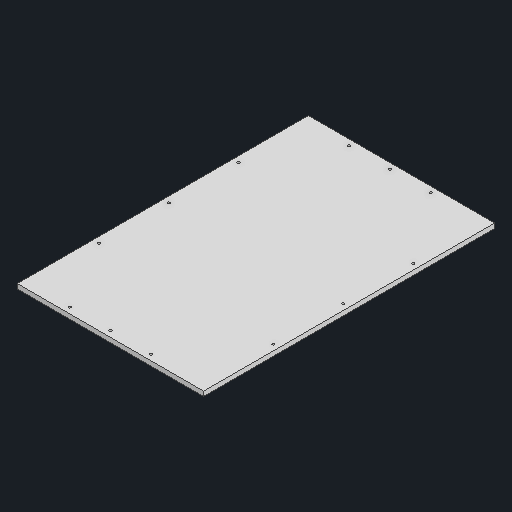
# Autodesk Inventor part: TeflonPlate
Saved by Autodesk Inventor 2027 (Build 310192060, 192F)
## iProperties
Created: 2026-06-12
Part Number: TeflonPlate
Material: Generic
Document SubType Name: Modeling
Designer: kw
Density: 1 g/cm^3
Appearance: Default
Author: kw
Autodesk Inventor part; units mm, degrees
ref_plane "YZ Plane" through (0, 0, 0) normal (1, 0, 0) x (0, 1, 0)
ref_plane "XZ Plane" through (0, 0, 0) normal (0, 1, 0) x (-1, 0, 0)
ref_plane "XY Plane" through (0, 0, 0) normal (0, 0, 1) x (1, 0, 0)
sketch "Sketch1" plane through (0, 0, 0) normal (0, 1, 0) x (-1, 0, 0)
  line L0 (0, 0) -> (-300, 0)
  line L1 (-300, 0) -> (-300, -500)
  line L2 (-300, -500) -> (0, -500)
  line L3 (0, -500) -> (0, 0)
  line L4 (-300, -500) -> (-320, -500)
  line L5 (-320, -500) -> (-320, 0)
  line L6 (-320, 0) -> (-300, 0)
  line L7 (-300, 0) -> (-300, -500)
  dimension "d101" = 300
  dimension "d102" = 500
  dimension "d110" = 20
  constraints: 16 end point, 4 parallel, 2 horizontal, 2 perpendicular
  measures "d101" distance of L2.end L1.end
  measures "d102" distance of L1.end L0.end
  measures "d110" distance of L5.end L6.end
extrude "Extrusion1" add sketch "Sketch1" along normal blind 8
sketch "Sketch4" plane through (0, 8, 0) normal (0, 1, 0) x (1, 0, 0)
  circle A0 centre (80, 490) radius 2.15 projected
  circle A1 centre (150, 490) radius 2.15 projected
  circle A2 centre (220, 490) radius 2.15 projected
  circle A3 centre (80, 10) radius 2.15 projected
  circle A4 centre (150, 10) radius 2.15 projected
  circle A5 centre (220, 10) radius 2.15 projected
  point P0 (0, 0)
hole "Hole1" at (80, 8, -490) at (150, 8, -490) at (220, 8, -490) at (80, 8, -10) at (150, 8, -10) at (220, 8, -10) direction (0, -1, 0) diameter 4.3 depth 8 clearance for "Socket Head Cap Screw ISO 4762" size "M4" standard "ISO"
sketch "Sketch5" plane through (0, 8, 0) normal (0, 1, 0) x (1, 0, 0)
  line L0 (10, 0) -> (10, 130)
  line L1 (0, 0) -> (320, 0) projected
  line L2 (10, 0) -> (140, 0) construction
  line L3 (10, 130) -> (10, 250)
  line L4 (10, 250) -> (10, 370)
  line L5 (10, 370) -> (10, 500)
  point P0 (310, 370)
  point P1 (310, 250)
  point P2 (310, 130)
  dimension "d111" = 130
  dimension "d112" = 90
  dimension "d113" = 120
  dimension "d114" = 120
  dimension "d115" = 130
  constraints: 10 end point, 3 point on line, 2 perpendicular, 1 horizontal
  measures "d111" distance of L0.start L0.end
  measures "d112" angle of L2 L0
  measures "d113" distance of L0.end L3.end
  measures "d114" distance of L3.end L4.end
  measures "d115" distance of L4.end L5.end
hole "Hole2" at (310, 8, -370) at (310, 8, -250) at (310, 8, -130) at (10, 8, -370) at (10, 8, -250) at (10, 8, -130) direction (0, -1, 0) diameter 4.3 end through all clearance for "Socket Head Cap Screw ISO 4762" size "M4" standard "ISO"
body "Solid1"
